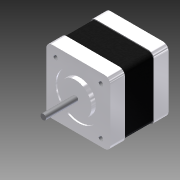
# Autodesk Inventor part: Nema17
Saved by Autodesk Inventor 2012 SP1 (Build 160190100, 190)
## iProperties
Created: 2012-03-17
Part Number: Nema17
Material: Default
Document SubType Name: Modeling
Designer: Matt
Density: 1 g/cm^3
Author: Matt
Autodesk Inventor part; units mm, degrees
ref_plane "YZ Plane" through (0, 0, 0) normal (1, 0, 0) x (0, 1, 0)
ref_plane "XZ Plane" through (0, 0, 0) normal (0, 1, 0) x (-1, 0, 0)
ref_plane "XY Plane" through (0, 0, 0) normal (0, 0, 1) x (1, 0, 0)
sketch "Sketch1" plane through (0, 0, 0) normal (0, 0, 1) x (1, 0, 0)
  line L0 (-8.2846, 3.8499) -> (34.0154, 3.8499)
  line L1 (34.0154, 3.8499) -> (34.0154, -38.4501)
  line L2 (34.0154, -38.4501) -> (-8.2846, -38.4501)
  line L3 (-8.2846, -38.4501) -> (-8.2846, 3.8499)
  circle A0 centre (12.8654, -17.3001) radius 11
  circle A1 centre (12.8654, -17.3001) radius 1.891
  circle A2 centre (12.8654, -17.3001) radius 15.5
  circle A3 centre (-2.6346, -32.8001) radius 1.5
  circle A4 centre (28.3654, -34.3001) radius 1.5
  circle A5 centre (28.3654, -1.8001) radius 1.5
  circle A6 centre (-2.6346, -1.8001) radius 1.5
  point P0 (0, 0)
  dimension "d0" = 42.3
  dimension "d1" = 42.3
  dimension "d2" = 22
  dimension "d3" = 31
  dimension "d4" = 3
  dimension "d5" = 3
  dimension "d6" = 3
  dimension "d7" = 3
  constraints: 8 end point, 7 centre point, 2 coincident, 2 parallel, 1 horizontal, 1 perpendicular
  measures "d0" distance of L1.end L2.end
  measures "d1" distance of L0.end L1.end
  measures "d2" diameter of A0
  measures "d3" diameter of A2
  measures "d4" diameter of A3
  measures "d5" diameter of A4
  measures "d6" diameter of A5
  measures "d7" diameter of A6
extrude "Extrusion1" add sketch "Sketch1" along normal blind 40 contours L0 L1 L2 L3 | A0 | A1 | A2
fillet "Fillet1" radius 3.175 4 edges at (34.0154, 3.8499, 20) (-8.2846, 3.8499, 20) (34.0154, -38.4501, 20) (-8.2846, -38.4501, 20)
sketch "Sketch2" plane through (0, 0, 40) normal (0, 0, 1) x (1, 0, 0)
  circle A0 centre (12.8654, -17.3001) radius 15.5 projected
  circle A1 centre (12.8654, -17.3001) radius 1.891 projected
  circle A2 centre (12.8654, -17.3001) radius 11 projected
  point P0 (0, 0)
extrude "Extrusion2" add sketch "Sketch2" along normal blind 2 contours A2
sketch "Sketch3" plane through (0, 0, 40) normal (0, 0, 1) x (1, 0, 0)
  circle A0 centre (12.8654, -17.3001) radius 11 projected
  circle A1 centre (12.8654, -17.3001) radius 15.5 projected
  point P0 (0, 0)
extrude "Extrusion3" cut sketch "Sketch3" against normal blind 1
sketch "Sketch4" plane through (12.8654, -17.3001, 42) normal (0, 0, 1) x (1, 0, 0)
  circle A0 centre (0, 0) radius 1.891 projected
  point P0 (-12.8654, 17.3001)
extrude "Extrusion4" add sketch "Sketch4" along normal blind 22
sketch "Sketch5" plane through (0, 0, 40) normal (0, 0, 1) x (1, 0, 0)
  arc A0 (-8.2846, -35.2751) -> (-5.1096, -38.4501) centre (-5.1096, -35.2751) ccw projected
  line L0 (30.8404, -38.4501) -> (-5.1096, -38.4501) projected
  arc A1 (30.8404, -38.4501) -> (34.0154, -35.2751) centre (30.8404, -35.2751) ccw projected
  line L1 (34.0154, 0.6749) -> (34.0154, -35.2751) projected
  arc A2 (34.0154, 0.6749) -> (30.8404, 3.8499) centre (30.8404, 0.6749) ccw projected
  line L2 (-5.1096, 3.8499) -> (30.8404, 3.8499) projected
  arc A3 (-5.1096, 3.8499) -> (-8.2846, 0.6749) centre (-5.1096, 0.6749) ccw projected
  line L3 (-8.2846, -35.2751) -> (-8.2846, 0.6749) projected
  arc A4 (34.7866, 0.6749) -> (30.8404, 4.6211) centre (30.8404, 0.6749) ccw
  line L4 (34.7866, 0.6749) -> (34.7866, -35.2751)
  arc A5 (30.8404, -39.2213) -> (34.7866, -35.2751) centre (30.8404, -35.2751) ccw
  line L5 (30.8404, -39.2213) -> (-5.1096, -39.2213)
  arc A6 (-9.0558, -35.2751) -> (-5.1096, -39.2213) centre (-5.1096, -35.2751) ccw
  line L6 (-9.0558, -35.2751) -> (-9.0558, 0.6749)
  arc A7 (-5.1096, 4.6211) -> (-9.0558, 0.6749) centre (-5.1096, 0.6749) ccw
  line L7 (-5.1096, 4.6211) -> (30.8404, 4.6211)
  point P0 (0, 0)
  constraints: 8 end point, 8 point on circle, 4 centre point, 7 other
extrude "Extrusion5" add sketch "Sketch5" against normal blind 10
sketch "Sketch6" plane through (0, 0, 0) normal (0, 0, -1) x (-1, 0, 0)
  arc A0 (5.1096, -38.4501) -> (8.2846, -35.2751) centre (5.1096, -35.2751) ccw projected
  line L0 (8.2846, -35.2751) -> (8.2846, 0.6749) projected
  arc A1 (8.2846, 0.6749) -> (5.1096, 3.8499) centre (5.1096, 0.6749) ccw projected
  line L1 (5.1096, 3.8499) -> (-30.8404, 3.8499) projected
  arc A2 (-30.8404, 3.8499) -> (-34.0154, 0.6749) centre (-30.8404, 0.6749) ccw projected
  line L2 (-34.0154, 0.6749) -> (-34.0154, -35.2751) projected
  arc A3 (-34.0154, -35.2751) -> (-30.8404, -38.4501) centre (-30.8404, -35.2751) ccw projected
  line L3 (-30.8404, -38.4501) -> (5.1096, -38.4501) projected
  line L4 (8.9119, 0.6749) -> (8.9119, -35.2751)
  arc A4 (5.1096, -39.0774) -> (8.9119, -35.2751) centre (5.1096, -35.2751) ccw
  line L5 (5.1096, -39.0774) -> (-30.8404, -39.0774)
  arc A5 (-34.6427, -35.2751) -> (-30.8404, -39.0774) centre (-30.8404, -35.2751) ccw
  line L6 (-34.6427, -35.2751) -> (-34.6427, 0.6749)
  arc A6 (-30.8404, 4.4772) -> (-34.6427, 0.6749) centre (-30.8404, 0.6749) ccw
  line L7 (-30.8404, 4.4772) -> (5.1096, 4.4772)
  arc A7 (8.9119, 0.6749) -> (5.1096, 4.4772) centre (5.1096, 0.6749) ccw
  point P0 (0, 0)
  constraints: 8 end point, 8 point on circle, 4 centre point, 7 other
extrude "Extrusion6" add sketch "Sketch6" against normal blind 10
body "Solid1"
